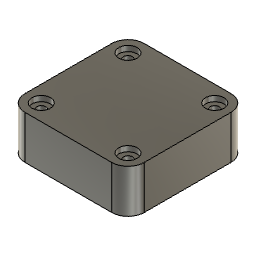
suporte_lidar (Autodesk Fusion 360 design; units mm, degrees)
Autodesk Fusion 360 part; units mm, degrees
sketch "Esboço1" plane through (0, 0, 0) normal (0, 0, 1) x (1, 0, 0)
  line L0 (15, 0) -> (95, 0)
  line L1 (110, 15) -> (110, 95)
  line L2 (95, 110) -> (15, 110)
  line L3 (0, 95) -> (0, 15)
  circle A0 centre (15, 15) radius 4.1
  arc A1 (15, 110) -> (0, 95) centre (15, 95) ccw
  circle A2 centre (15, 95) radius 4.1
  arc A3 (110, 95) -> (95, 110) centre (95, 95) ccw
  arc A4 (95, 0) -> (110, 15) centre (95, 15) ccw
  arc A5 (0, 15) -> (15, 0) centre (15, 15) ccw
  circle A6 centre (95, 15) radius 4.1
  circle A7 centre (95, 95) radius 4.1
  point P0 (110, 0)
  point P1 (0, 110)
  dimension "d1" = 110
  dimension "d2" = 110
  dimension "d3" = 8.2
  dimension "d4" = 15
  dimension "d5" = 8.2
  dimension "d6" = 15
  dimension "d7" = 8.2
  dimension "d8" = 8.2
  constraint horizontal L0
  constraint vertical L1
  constraint horizontal L2
  constraint vertical L3
  constraint coincident P1 L2
  constraint coincident P1 L3
  constraint tangent L2 A1
  constraint tangent L3 A1
  constraint concentric A1 A2
  constraint tangent L1 A3
  constraint tangent L2 A3
  constraint coincident P0 L0
  constraint coincident P0 L1
  constraint tangent L0 A4
  constraint tangent L1 A4
  constraint equal A3 A4
  constraint coincident origin L0
  constraint coincident origin L3
  constraint tangent L0 A5
  constraint tangent L3 A5
  constraint equal A3 A5
  constraint coincident A0.centre A5.centre
  constraint concentric A4 A6
  constraint concentric A3 A7
  measures "d1" distance of origin P0
  measures "d2" distance of origin P1
  measures "d3" diameter of A0
  measures "d4" radius of A1
  measures "d5" diameter of A2
  measures "d6" radius of A3
  measures "d7" diameter of A6
  measures "d8" diameter of A7
extrude "Extrusão1" add sketch "Esboço1" along normal blind 40
sketch "Esboço2" plane through (0, 0, 40) normal (0, 0, 1) x (-1, 0, 0)
  circle A0 centre (-15, -95) radius 4.1
  circle A1 centre (-95, -15) radius 4.1
  circle A2 centre (-95, -95) radius 4.1
  circle A3 centre (-15, -15) radius 4.1
  arc A4 (0, -15) -> (-15, 0) centre (-15, -15) ccw
  line L0 (-15, 0) -> (-95, 0)
  arc A5 (-95, 0) -> (-110, -15) centre (-95, -15) ccw
  line L1 (-110, -15) -> (-110, -95)
  arc A6 (-110, -95) -> (-95, -110) centre (-95, -95) ccw
  line L2 (-95, -110) -> (-15, -110)
  arc A7 (-15, -110) -> (0, -95) centre (-15, -95) ccw
  line L3 (0, -95) -> (0, -15)
  circle A8 centre (-15, -15) radius 8.5
  circle A9 centre (-15, -15) radius 8.5
  circle A10 centre (-15, -95) radius 8.5
  circle A11 centre (-95, -95) radius 8.5
  circle A12 centre (-95, -15) radius 8.5
  dimension "d11" = 17
  dimension "d12" = 17
  dimension "d13" = 17
  dimension "d14" = 17
  dimension "d15" = 17
  constraint concentric A3 A8
  constraint concentric A0 A10
  constraint concentric A2 A11
  constraint concentric A1 A12
  measures "d11" diameter of A8
  measures "d12" diameter of A9
  measures "d13" diameter of A10
  measures "d14" diameter of A11
  measures "d15" diameter of A12
extrude "Extrusão2" cut sketch "Esboço2" against normal blind 5 contours A8 A9 | A10 | A11 | A12
